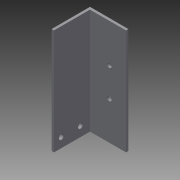
# Autodesk Inventor part: 2x2 angle vertical left
Saved by Autodesk Inventor 2015 SP1 (Build 190203100, 203)
## iProperties
Created: 2015-01-16
Part Number: 2x2 angle vertical left
Material: Generic
Document SubType Name: Modeling
Designer: Jarod
Density: 1 g/cm^3
Appearance: Default
Author: Jarod
Autodesk Inventor part; units mm, degrees
ref_plane "YZ Plane" through (0, 0, 0) normal (1, 0, 0) x (0, 1, 0)
ref_plane "XZ Plane" through (0, 0, 0) normal (0, 1, 0) x (-1, 0, 0)
ref_plane "XY Plane" through (0, 0, 0) normal (0, 0, 1) x (1, 0, 0)
sketch "Sketch1" plane through (0, 0, 0) normal (0, 1, 0) x (-1, 0, 0)
  line L0 (0, 0) -> (-3.175, 0)
  line L1 (-3.175, 0) -> (-3.175, 50.8)
  line L2 (-3.175, 50.8) -> (0, 50.8)
  line L3 (0, 50.8) -> (0, 0)
  line L4 (0, 0) -> (-50.8, 0)
  line L5 (-50.8, 0) -> (-50.8, 3.175)
  line L6 (-50.8, 3.175) -> (0, 3.175)
  line L7 (0, 3.175) -> (0, 0)
  dimension "d0" = 3.175
  dimension "d1" = 50.8
  dimension "d2" = 50.8
  dimension "d3" = 3.175
  constraints: 16 end point, 4 parallel, 2 horizontal, 2 perpendicular
  measures "d0" distance of L1.end L2.end
  measures "d1" distance of L0.end L1.end
  measures "d2" distance of L5.end L6.end
  measures "d3" distance of L4.end L5.end
extrude "Extrusion1" add sketch "Sketch1" against normal blind 139.7
sketch "Sketch3" plane through (0, 0, 0) normal (-1, 0, 0) x (0, 0, 1)
  line L0 (0, 0) -> (50.8, 0) projected
  line L1 (0, 0) -> (0, -139.7) projected
  line L2 (50.8, -139.7) -> (0, -139.7) projected
  line L3 (50.8, 0) -> (50.8, -139.7) projected
  point P0 (15.875, -127)
  point P1 (41.275, -127)
  dimension "d17" = 9.525
  dimension "d18" = 12.7
  dimension "d19" = 12.7
  dimension "d20" = 15.875
  measures "d17" distance from line of L3 point (41.275, -127)
  measures "d18" distance from line of L2 point (41.275, -127)
  measures "d19" distance from line of L2 point (15.875, -127)
  measures "d20" distance from line of L1 point (15.875, -127)
hole "Hole2" at (0, -127, 15.875) at (0, -127, 41.275) direction (1, 0, 0) diameter 6.35 end through all
sketch "Sketch4" plane through (50.8, 0, 0) normal (0, 0, -1) x (-1, 0, 0)
  line L0 (50.8, -139.7) -> (0, -139.7) projected
  line L1 (50.8, 0) -> (50.8, -139.7) projected
  line L2 (0, 0) -> (50.8, 0) projected
  line L3 (0, 0) -> (0, -139.7) projected
  point P0 (22.225, -63.5)
  point P1 (22.225, -101.6)
  dimension "d28" = 28.575
  dimension "d29" = 28.575
  dimension "d30" = 63.5
  dimension "d31" = 101.6
  measures "d28" distance from line of point (22.225, -63.5) L1
  measures "d29" distance from line of L1 point (22.225, -101.6)
  measures "d30" distance from line of L2 point (22.225, -63.5)
  measures "d31" distance from line of point (22.225, -101.6) L2
hole "Hole3" at (28.575, -63.5, 0) at (28.575, -101.6, 0) direction (0, 0, 1) diameter 6.35 end through all
sketch "Sketch5" plane through (0, 0, 0) normal (0, 1, 0) x (1, 0, 0)
  line L0 (0, 0) -> (0, -50.8) projected
  line L1 (0, -50.8) -> (3.175, -50.8) projected
  line L2 (3.175, -50.8) -> (3.175, -3.175) projected
  line L3 (3.175, -3.175) -> (50.8, -3.175) projected
  line L4 (50.8, -3.175) -> (50.8, 0) projected
  line L5 (50.8, 0) -> (0, 0) projected
  line L6 (0, 0) -> (3.175, 0)
  line L7 (3.175, 0) -> (3.175, -50.8)
  line L8 (3.175, -50.8) -> (0, -50.8)
  line L9 (0, -50.8) -> (0, 0)
  constraints: 8 end point, 2 parallel, 1 horizontal, 1 perpendicular
extrude "Extrusion2" add sketch "Sketch5" along normal blind 50.8 contours L5 L7 L2 L1 L0
sketch "Sketch6" plane through (0, 0, 0) normal (0, 1, 0) x (1, 0, 0)
  line L0 (3.175, 0) -> (3.175, -3.175) projected
  line L1 (3.175, -3.175) -> (50.8, -3.175) projected
  line L2 (50.8, -3.175) -> (50.8, 0) projected
  line L3 (50.8, 0) -> (3.175, 0) projected
  line L4 (50.8, 0) -> (28.575, 0)
  line L5 (28.575, 0) -> (28.575, -3.175)
  line L6 (28.575, -3.175) -> (50.8, -3.175)
  line L7 (50.8, -3.175) -> (50.8, 0)
  point P0 (0, 0)
  dimension "d41" = 22.225
  constraints: 8 end point, 2 parallel, 1 horizontal, 1 perpendicular, 1 point on line
  measures "d41" distance of L6.end L5.end
extrude "Extrusion3" cut sketch "Sketch6" against normal blind 50.8 contours L3 L2 L1 L5
sketch "Sketch7" plane through (0, -139.7, 0) normal (-1, 0, 0) x (0, 0, 1)
  circle A0 centre (15.875, 12.7) radius 3.175 projected
  circle A1 centre (41.275, 12.7) radius 3.175 projected
  line L0 (0, 190.5) -> (0, 0) projected
  line L1 (50.8, 0) -> (0, 0) projected
  line L2 (50.8, 0) -> (50.8, 190.5) projected
  line L3 (0, 190.5) -> (50.8, 190.5) projected
  point P0 (0, 139.7)
  point P1 (12.7, 177.8)
  point P2 (38.1, 177.8)
  point P3 (38.1, 152.4)
  point P4 (12.7, 152.4)
  dimension "d44" = 12.7
  dimension "d45" = 38.1
  dimension "d46" = 38.1
  dimension "d47" = 12.7
  dimension "d48" = 12.7
  dimension "d49" = 12.7
  dimension "d50" = 12.7
  dimension "d51" = 12.7
  measures "d44" distance from line of L0 point (12.7, 152.4)
  measures "d45" distance from line of L3 point (12.7, 152.4)
  measures "d46" distance from line of L3 point (38.1, 152.4)
  measures "d47" distance from line of L2 point (38.1, 152.4)
  measures "d48" distance from line of L2 point (38.1, 177.8)
  measures "d49" distance from line of L3 point (38.1, 177.8)
  measures "d50" distance from line of L3 point (12.7, 177.8)
  measures "d51" distance from line of L0 point (12.7, 177.8)
hole "Hole4" at (0, 38.1, 12.7) at (0, 38.1, 38.1) at (0, 12.7, 38.1) at (0, 12.7, 12.7) direction (1, 0, 0) diameter 6.35 end through all
body "Solid1"
